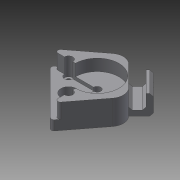
# Autodesk Inventor part: leveling clip
Saved by Autodesk Inventor 2014 (Build 180170000, 170)
## iProperties
Created: 2016-05-11
Part Number: leveling clip
Material: Generic
Document SubType Name: Modeling
Designer: eric.parent
Density: 1 g/cm^3
Appearance: Default
Author: eric.parent
Autodesk Inventor part; units mm, degrees
ref_plane "YZ Plane" through (0, 0, 0) normal (1, 0, 0) x (0, 1, 0)
ref_plane "XZ Plane" through (0, 0, 0) normal (0, 1, 0) x (-1, 0, 0)
sketch "Sketch1" plane through (0, 0, 0) normal (0, 0, 1) x (1, 0, 0)
  line L0 (202, 202) -> (202, 0) construction
  line L1 (0, 202) -> (202, 202) construction
  arc A0 (206.2012, 222.0831) -> (193.0425, 222.9456) centre (199.1301, 215.012) ccw projected
  arc A1 (222.9456, 193.0425) -> (222.0831, 206.2012) centre (215.012, 199.1301) ccw projected
  line L2 (206.2012, 222.0831) -> (222.0831, 206.2012)
  line L3 (193.0425, 222.9456) -> (165.7457, 202)
  line L4 (202, 165.7457) -> (222.9456, 193.0425)
  line L5 (165.7457, 202) -> (202, 165.7457)
  point P0 (0, 0)
  constraints: 8 end point, 3 tangent, 2 point on line, 1 parallel
extrude "Extrusion3" add sketch "Sketch1" along normal blind 19
sketch "Sketch3" plane through (0, 0, 19) normal (0, 0, 1) x (1, 0, 0)
  line L0 (165.7457, 202) -> (202, 202)
  line L1 (202, 202) -> (202, 165.7457)
  line L2 (165.7457, 202) -> (202, 165.7457)
  point P0 (0, 0)
  constraints: 6 end point, 1 horizontal, 1 perpendicular
extrude "Extrusion4" cut sketch "Sketch3" against normal blind 11.5
sketch "Sketch5" plane through (0, 0, 19) normal (0, 0, 1) x (1, 0, 0)
  line L0 (222.0831, 206.2012) -> (206.2012, 222.0831) construction
  line L1 (214.1421, 214.1421) -> (134.2284, 134.2284) construction
  line L2 (202, 165.7457) -> (165.7457, 202) construction
  circle A0 centre (190.9439, 190.9439) radius 6
  point P0 (0, 0)
  dimension "d25" = 12
  dimension "d26" = 10
  constraints: 2 end point, 1 centre point, 1 midpoint, 1 perpendicular, 1 point on line
  measures "d25" diameter of A0
  measures "d26" distance from line of L2 A0.centre
extrude "Extrusion6" cut sketch "Sketch5" against normal through all
sketch "Sketch6" plane through (0, 0, 19) normal (0, 0, 1) x (1, 0, 0)
  circle A0 centre (202, 202) radius 2.75
  point P0 (0, 0)
  dimension "d27" = 5.5
  constraints: 1 centre point, 1 coincident
  measures "d27" diameter of A0
extrude "Extrusion7" cut sketch "Sketch6" against normal through all
sketch "Sketch7" plane through (0, 0, 19) normal (0, 0, 1) x (1, 0, 0)
  arc A0 (202, 199.25) -> (199.25, 202) centre (202, 202) ccw construction
  circle A1 centre (202, 202) radius 16.75
  point P0 (0, 0)
  dimension "d30" = 33.5
  constraints: 1 centre point, 1 coincident
  measures "d30" diameter of A1
extrude "Extrusion8" cut sketch "Sketch7" against normal blind 9
sketch "Sketch8" plane through (0, 0, 19) normal (0, 0, 1) x (1, 0, 0)
  line L0 (202, 185.25) -> (202, 165.7457) construction
  circle A0 centre (190.9439, 190.9439) radius 6 construction
  line L1 (202, 165.7457) -> (165.7457, 202) construction
  line L2 (163.0953, 218.7925) -> (219.2426, 162.6452) construction
  circle A1 centre (202, 179.8878) radius 1.65
  point P0 (0, 0)
  dimension "d33" = 3.3
  constraints: 3 point on line, 2 end point, 1 centre point, 1 parallel
  measures "d33" diameter of A1
extrude "Extrusion9" cut sketch "Sketch8" against normal through all
sketch "Sketch9" plane through (0, 0, 19) normal (0, 0, 1) x (1, 0, 0)
  arc A0 (202, 178.2378) -> (202, 181.5378) centre (202, 179.8878) ccw construction
  circle A1 centre (202, 179.8878) radius 3.25
  point P0 (0, 0)
  dimension "d36" = 6.5
  constraints: 1 centre point, 1 coincident
  measures "d36" diameter of A1
extrude "Extrusion10" cut sketch "Sketch9" against normal blind 14
ref_plane "Work Plane1" through (183.8728, 183.8728, 7.5) normal (0.7071068, -0.7071068, 0) x (0, 0, -1)
mirror "Mirror1" about plane through (183.8728, 183.8728, 7.5) normal (0.7071068, -0.7071068, 0) of "Extrusion9", "Extrusion10"
fillet "Fillet6" radius 2 4 edges at (165.7457, 202, 13.25) (165.7457, 202, 3.75) (202, 165.7457, 13.25) (202, 165.7457, 3.75)
sketch "Sketch10" plane through (0, 0, 10) normal (0, 0, 1) x (1, 0, 0)
  line L0 (202, 185.25) -> (202, 199.25) projected
  arc A0 (202, 185.25) -> (185.25, 202) centre (202, 202) ccw projected
  line L1 (199.25, 202) -> (185.25, 202) projected
  arc A1 (202, 199.25) -> (199.25, 202) centre (202, 202) ccw projected
  point P0 (0, 0)
sketch "Sketch11" plane through (183.8728, 183.8728, 7.5) normal (0.7071068, -0.7071068, 0) x (0, 0, -1)
  line L0 (7.5, 42.8073) -> (-11.5, 42.8073) construction
  line L1 (7.5, 34.1125) -> (7.5, 42.8073) construction
  line L2 (7.5, 42.8073) -> (7.5, 56.3323)
  line L3 (7.5, 56.3323) -> (-7.5, 56.3323)
  line L4 (-7.5, 56.3323) -> (-7.5, 52.3323)
  line L5 (-7.5, 52.3323) -> (3.5, 52.3323)
  line L6 (3.5, 52.3323) -> (3.5, 42.8073)
  line L7 (3.5, 42.8073) -> (7.5, 42.8073)
  line L8 (-11.5, 5.8414) -> (-11.5, 34.1125) projected
  point P0 (7.5, -260.0355)
  dimension "d42" = 4
  dimension "d43" = 4
  dimension "d44" = 9.525
  dimension "d47" = 15
  constraints: 12 end point, 2 collinear, 2 parallel, 2 perpendicular, 1 point on line
  measures "d42" distance between parallel lines of L2 L6
  measures "d43" distance between parallel lines of L3 L5
  measures "d44" distance of L5.end L6.end
  measures "d47" distance between parallel lines of L2 L4
extrude "Extrusion11" add sketch "Sketch11" along normal up to surface (11.2302 mm away)
mirror "Mirror2" about plane through (183.8728, 183.8728, 7.5) normal (0.7071068, -0.7071068, 0) of "Extrusion11"
chamfer "Chamfer1" distance 2 angle 45 3 edges at (214.1421, 214.1421, 4) (220.8773, 220.8773, 4) (223.7058, 223.7058, 0)
sketch "Sketch12" plane through (215.7648, 231.6467, 2) normal (0.7071068, 0.7071068, 0) x (-0.7071068, 0.7071068, 0)
  line L0 (0, 13) -> (-22.4605, 13) construction
  line L1 (-13.7302, 11) -> (-8.7302, 11)
  line L2 (-8.7302, 11) -> (-8.7302, 9)
  line L3 (-8.7302, 9) -> (-13.7302, 9)
  line L4 (-13.7302, 9) -> (-13.7302, 11)
  line L5 (-11.2302, -2) -> (-11.2302, 26.4144) construction
  line L6 (-47.3365, 10) -> (30.7363, 10) construction
  dimension "d51" = 2
  dimension "d52" = 5
  dimension "d53" = 3
  constraints: 12 end point, 3 parallel, 2 perpendicular, 1 horizontal, 2 other
  measures "d51" distance of L3.end L1.start
  measures "d52" distance of L1.start L1.end
  measures "d53" distance between parallel lines of L0 L6
extrude "Extrusion12" cut sketch "Sketch12" against normal up to surface (4 mm away)
sketch "Sketch13" plane through (227.4041, 211.5221, 4) normal (0, 0, 1) x (0.7071068, 0.7071068, 0)
  line L0 (-7.525, 0) -> (-7.525, 22.4605) construction
  line L1 (5.9252, 11.2302) -> (-17.6111, 11.2302) construction
  line L2 (-7.525, 13.7302) -> (-5.525, 13.7302)
  line L3 (-5.525, 13.7302) -> (-5.525, 8.7302)
  line L4 (-5.525, 8.7302) -> (-7.525, 8.7302)
  line L5 (-7.525, 8.7302) -> (-7.525, 13.7302)
  point P0 (-310.3677, 11.2302)
  dimension "d56" = 2
  dimension "d57" = 5
  constraints: 10 end point, 2 parallel, 2 perpendicular, 1 horizontal, 1 point on line, 1 other
  measures "d56" distance of L3.end L4.end
  measures "d57" distance of L2.end L3.end
extrude "Extrusion13" cut sketch "Sketch13" against normal up to surface (4 mm away)
chamfer "Chamfer2" distance 2 angle 45 1 edges at (223.7058, 223.7058, 15)
body "Solid2"
